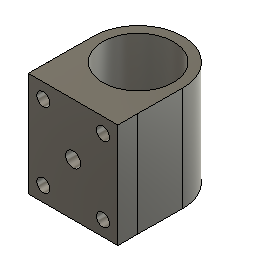
Caster Foot Keyboard Stand (Autodesk Fusion 360 design; units mm, degrees)
Autodesk Fusion 360 part; units mm, degrees
sketch "Skizze1" plane through (0, 0, 0) normal (0, 1, 0) x (1, 0, 0)
  circle A0 centre (0, 0) radius 14.2
  line L0 (-18.1535, -18) -> (17.8465, -18)
  line L1 (17.8465, -18) -> (17.8465, -26)
  line L2 (17.8465, -26) -> (-18.1535, -26)
  line L3 (-18.1535, -26) -> (-18.1535, -18)
  line L4 (-18.1535, -18) -> (17.8465, -26) construction
  line L5 (17.8465, -18) -> (-18.1535, -26) construction
  circle A1 centre (0, 0) radius 18
  line L6 (-18.1535, -18) -> (-17.9994, 0.1529)
  line L7 (17.8465, -18) -> (17.9993, -0.1542)
  point P0 (-0.1535, -22)
  dimension "d1" = 28.4
  dimension "d2" = 36
  dimension "d3" = 8
  dimension "d4" = 36
  constraint coincident A0.centre A1.centre
  constraint horizontal L0
  constraint perpendicular L0 L1
  constraint parallel L0 L2
  constraint parallel L1 L3
  constraint coincident L4 P0
  constraint coincident L5 P0
  constraint tangent L0 A1
  constraint coincident A1 L6.end
  constraint tangent A1 L6
  constraint coincident A1 L7.end
  constraint tangent A1 L7
  measures "d1" diameter of A0
  measures "d2" distance of L1.end L2.end
  measures "d3" distance of L0.end L1.end
  measures "d4" diameter of A1
extrude "Extrusion1" add sketch "Skizze1" along normal blind 42
sketch "Skizze3" plane through (0, 0, 26) normal (0, 0, 1) x (1, 0, 0)
  line L0 (-18.1535, 0) -> (17.8465, 0)
  line L1 (17.8465, 0) -> (17.8465, 42)
  line L2 (17.8465, 42) -> (-18.1535, 42)
  line L3 (-18.1535, 42) -> (-18.1535, 0)
  circle A0 centre (-12.1535, 36) radius 2.6
  circle A1 centre (11.8465, 36) radius 2.6
  circle A2 centre (-12.1535, 6) radius 2.6
  circle A3 centre (11.8465, 6) radius 2.6
  dimension "d7" = 5.2
  dimension "d8" = 5.2
  dimension "d9" = 5.2
  dimension "d10" = 5.2
  dimension "d11" = 24
  dimension "d12" = 24
  dimension "d13" = 30
  dimension "d14" = 30
  dimension "d15" = 6
  dimension "d16" = 6
  dimension "d17" = 6
  measures "d7" diameter of A0
  measures "d8" diameter of A1
  measures "d9" diameter of A2
  measures "d10" diameter of A3
  measures "d11" distance of A0.centre A1.centre
  measures "d12" horizontal distance of A2.centre A3.centre
  measures "d13" vertical distance of A0.centre A2.centre
  measures "d14" vertical distance of A1.centre A3.centre
  measures "d15" distance of L1 A3.centre
  measures "d16" distance of L0 A3.centre
  measures "d17" distance of L1 A1.centre
extrude "Extrusion2" cut sketch "Skizze3" against normal blind 14 contours A0 | A1 | A2 | A3
sketch "Skizze4" plane through (0, 0, 26) normal (0, 0, 1) x (1, 0, 0)
  circle A0 centre (-12.1535, 6) radius 2.6
  circle A1 centre (11.8465, 36) radius 2.6
  circle A2 centre (-12.1535, 36) radius 2.6
  circle A3 centre (11.8465, 6) radius 2.6
  line L0 (-18.1535, 0) -> (17.8465, 0)
  line L1 (17.8465, 0) -> (17.8465, 42)
  line L2 (17.8465, 42) -> (-18.1535, 42)
  line L3 (-18.1535, 42) -> (-18.1535, 0)
  line L4 (-18.1535, 0) -> (17.8465, 42) construction
  line L5 (17.8465, 0) -> (-18.1535, 42) construction
  circle A4 centre (-0.1535, 21) radius 3
  circle A5 centre (-0.1535, 21) radius 2.05
  dimension "d20" = 6
  dimension "d21" = 4.1
  constraint coincident L0.start L3.end
  constraint coincident L1.end L2.start
  constraint coincident L0.end L1.start
  constraint coincident L2.end L3.start
  constraint midpoint L5 A4.centre
  constraint concentric A4 A5
  measures "d20" diameter of A4
  measures "d21" diameter of A5
extrude "Extrusion3" cut sketch "Skizze4" against normal blind 16 contours A5
extrude "Extrusion4" cut sketch "Skizze4" against normal blind 5.5 contours A4
equation "d8 = d7"
equation "d9 = d7"
equation "d10 = d7"
equation "d15 = ( ( 36 - 24 ) / 2 ) * 1 mm"
equation "d16 = ( ( 42 - 30 ) / 2 ) * 1 mm"
equation "d17 = d15"
named bodies: "Caster Foot Keyboard"
